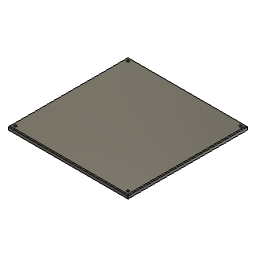
lid v1 (Autodesk Fusion 360 design; units mm, degrees)
Autodesk Fusion 360 part; units mm, degrees
sketch "Sketch1" plane through (0, 0, 0) normal (0, 1, 0) x (1, 0, 0)
  line L0 (0, 0) -> (172, 0)
  line L1 (172, 0) -> (172, -172)
  line L2 (172, -172) -> (0, -172)
  line L3 (0, -172) -> (0, 0)
  dimension "d1" = 172
  dimension "d2" = 172
  constraint horizontal L0
  constraint vertical L1
  constraint horizontal L2
  constraint vertical L3
  constraint coincident L0.start L3.end
  measures "d1" distance of L0.start L0.end
  measures "d2" distance of L0.start L2.end
extrude "Extrude1" add sketch "Sketch1" along normal blind 5
sketch "Sketch2" plane through (0, 5, 0) normal (0, 1, 0) x (-1, 0, 0)
  line L0 (0, 172) -> (-172, 172)
  line L1 (-172, 172) -> (-172, 0)
  line L2 (-172, 0) -> (0, 0)
  line L3 (0, 0) -> (0, 172)
  line L4 (0, 0) -> (-4.9497, 4.9497)
  line L5 (0, 0) -> (-7, 0) construction
  line L6 (-172, 172) -> (-167.0503, 167.0503)
  line L7 (-172, 172) -> (-165, 172) construction
  line L8 (-4.9497, 4.9497) -> (-167.0503, 4.9497)
  line L9 (-167.0503, 4.9497) -> (-167.0503, 167.0503)
  line L10 (-167.0503, 167.0503) -> (-4.9497, 167.0503)
  line L11 (-4.9497, 167.0503) -> (-4.9497, 4.9497)
  dimension "d5" = 45
  dimension "d6" = 7
  dimension "d7" = 45
  dimension "d8" = 7
  constraint horizontal L5
  constraint coincident L2.end L3.start
  constraint horizontal L7
  constraint coincident L0.end L1.start
  constraint horizontal L8
  constraint vertical L9
  constraint horizontal L10
  constraint vertical L11
  measures "d5" angle of L4 L5
  measures "d6" distance of L2.end L4.end
  measures "d7" angle of L6 L7
  measures "d8" distance of L0.end L6.end
hole "Hole1" at (4.9497, 5, 4.9497) at (167.0503, 5, 4.9497) at (167.0503, 5, 167.0503) at (4.9497, 5, 167.0503) direction (0, -1, 0) diameter 3.5 depth 9 tip angle 180
fillet "Fillet1" radius 1 4 edges at (0, 5, 86) (86, 5, 0) (172, 5, 86) (86, 5, 172)
